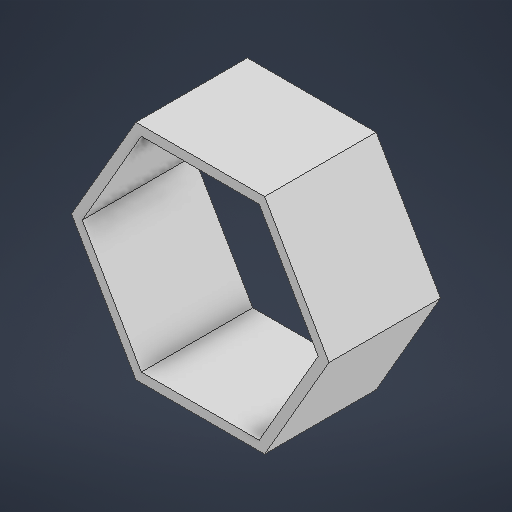
# Autodesk Inventor part: tolerance_test
Saved by Autodesk Inventor 2026.2 (Build 302298000, 298)
## iProperties
Created: 2026-04-15
Part Number: tolerance_test
Material: Generic
Document SubType Name: Modeling
Designer: cbast
Density: 1 g/cm^3
Appearance: Default
Author: cbast
Autodesk Inventor part; units mm, degrees
ref_plane "YZ Plane" through (0, 0, 0) normal (1, 0, 0) x (0, 1, 0)
ref_plane "XZ Plane" through (0, 0, 0) normal (0, 1, 0) x (-1, 0, 0)
ref_plane "XY Plane" through (0, 0, 0) normal (0, 0, 1) x (1, 0, 0)
sketch "Sketch1" plane through (0, 0, 0) normal (0, 0, 1) x (1, 0, 0)
  line L0 (0, 0) -> (17.0068, 0) construction
  line L1 (-2.6443, 4.5801) -> (-5.2887, 0)
  line L2 (-5.2887, 0) -> (-2.6443, -4.5801)
  line L3 (-2.6443, -4.5801) -> (2.6443, -4.5801)
  line L4 (2.6443, -4.5801) -> (5.2887, 0)
  line L5 (5.2887, 0) -> (2.6443, 4.5801)
  line L6 (2.6443, 4.5801) -> (-2.6443, 4.5801)
  line L7 (2.8867, 4.9999) -> (5.7734, 0)
  line L8 (5.7734, 0) -> (2.8867, -4.9999)
  line L9 (2.8867, -4.9999) -> (-2.8867, -4.9999)
  line L10 (-2.8867, -4.9999) -> (-5.7734, 0)
  line L11 (-5.7734, 0) -> (-2.8867, 4.9999)
  line L12 (-2.8867, 4.9999) -> (2.8867, 4.9999)
  constraints: 26 end point, 2 coincident, 1 horizontal, 1 point on line, 13 other
extrude "Extrusion1" add sketch "Sketch1" along normal blind 5
body "Solid1"
